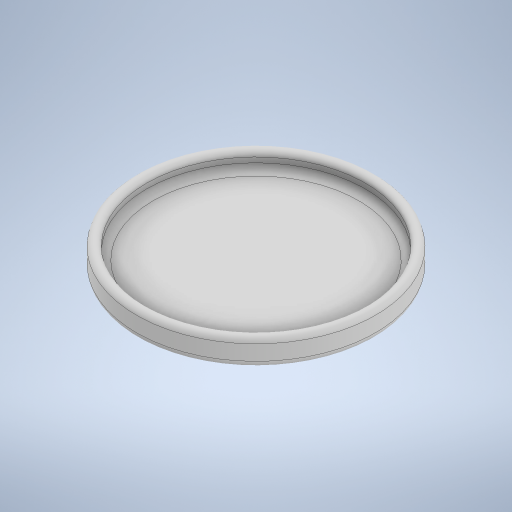
# Autodesk Inventor part: Orchid Coaster V2
Saved by Autodesk Inventor 2024 (Build 280153000, 153)
## iProperties
Created: 2024-02-28
Part Number: Orchid Coaster V2
Material: Generic
Document SubType Name: Modeling
Designer: haque
Density: 1 g/cm^3
Appearance: Default
Author: haque
Autodesk Inventor part; units mm, degrees
ref_plane "YZ Plane" through (0, 0, 0) normal (1, 0, 0) x (0, 1, 0)
ref_plane "XZ Plane" through (0, 0, 0) normal (0, 1, 0) x (-1, 0, 0)
ref_plane "XY Plane" through (0, 0, 0) normal (0, 0, 1) x (1, 0, 0)
sketch "Sketch1" plane through (0, 0, 0) normal (0, 1, 0) x (-1, 0, 0)
  circle A0 centre (0, 0) radius 32.5
  circle A1 centre (0, 0) radius 35.5
  dimension "d0" = 65
  dimension "d1" = 71
  constraints: 2 centre point, 2 coincident
  measures "d0" diameter of A0
  measures "d1" diameter of A1
extrude "Extrusion1" add sketch "Sketch1" along normal blind 8
extrude "Extrusion2" add sketch "Sketch1" along normal blind 3 contours A0
fillet "Fillet1" radius 2 2 edges at (35.5, 0, 0) (32.5, 3, 0)
fillet "Fillet2" radius 1.5 2 edges at (32.5, 8, 0) (35.5, 8, 0)
body "Solid1"
